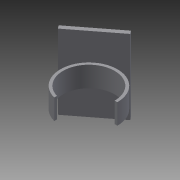
# Autodesk Inventor part: Clip
Saved by Autodesk Inventor 2015 (Build 190159000, 159)
## iProperties
Created: 2018-12-12
Part Number: Clip
Material: Generic
Document SubType Name: Modeling
Designer: 579494
Density: 1 g/cm^3
Appearance: Default
Author: 579494
Autodesk Inventor part; units mm, degrees
ref_plane "YZ Plane" through (0, 0, 0) normal (1, 0, 0) x (0, 1, 0)
ref_plane "XZ Plane" through (0, 0, 0) normal (0, 1, 0) x (-1, 0, 0)
ref_plane "XY Plane" through (0, 0, 0) normal (0, 0, 1) x (1, 0, 0)
sketch "Sketch1" plane through (0, 0, 0) normal (0, 0, 1) x (1, 0, 0)
  arc A0 (19, 0) -> (-5.2482, -18.2608) centre (0, 0) ccw
  line L0 (-5.2482, -18.2608) -> (-5.2482, -20.2608)
  line L1 (19, 0) -> (21, 0)
  arc A1 (21, 0) -> (-5.2482, -20.2608) centre (0.0001, 0.0728) ccw
  line L2 (-12.8316, 16.6965) -> (2.2089, 28.3061)
  line L3 (2.2089, 28.3061) -> (-12.8316, 16.6965)
  line L4 (-12.8316, 16.6965) -> (-27.8721, 5.0869)
  line L5 (-27.8721, 5.0869) -> (-29.7052, 7.4617)
  line L6 (-29.7052, 7.4617) -> (0.3758, 30.681)
  line L7 (0.3758, 30.681) -> (2.2089, 28.3061)
  point P0 (0, 0)
  dimension "d1" = 19
  dimension "d2" = 2
  dimension "d3" = 2
  dimension "d4" = 21
  dimension "d5" = 19
  dimension "d6" = 19
  dimension "d7" = 3
  constraints: 16 end point, 5 point on circle, 2 centre point, 2 perpendicular, 1 collinear, 1 horizontal, 1 point on line, 1 vertical
  measures "d1" radius of A0
  measures "d2" distance of L0.start L0.end
  measures "d3" distance of L1.start L1.end
  measures "d4" radius of A1
  measures "d5" distance of L2.start L2.end
  measures "d6" distance of L2.start L4.end
  measures "d7" distance of L4.end L5.end
extrude "Extrusion1" add sketch "Sketch1" along normal blind 15
sketch "Sketch2" plane through (0, 0, 0) normal (0, 0, -1) x (-1, 0, 0)
  line L0 (29.7052, 7.4617) -> (-0.3758, 30.681)
  line L1 (-0.3758, 30.681) -> (29.7052, 7.4617) projected
  line L2 (-0.3758, 30.681) -> (-2.2089, 28.3061)
  line L3 (-2.2089, 28.3061) -> (27.8721, 5.0869)
  line L4 (27.8721, 5.0869) -> (29.7052, 7.4617)
  point P0 (0, 0)
  constraints: 8 end point, 3 perpendicular, 1 collinear
extrude "Extrusion2" add sketch "Sketch2" along normal blind 20
sketch "Sketch3" plane through (0, 0, 15) normal (0, 0, 1) x (1, 0, 0)
  line L0 (0.3758, 30.681) -> (2.2089, 28.3061)
  line L1 (2.2089, 28.3061) -> (0.3758, 30.681) projected
  line L2 (2.2089, 28.3061) -> (-27.8721, 5.0869)
  line L3 (-27.8721, 5.0869) -> (-12.8316, 16.6965) projected
  line L4 (-27.8721, 5.0869) -> (-29.7052, 7.4617)
  line L5 (-29.7052, 7.4617) -> (0.3758, 30.681)
  point P0 (0, 0)
  constraints: 8 end point, 2 collinear, 2 perpendicular
extrude "Extrusion3" add sketch "Sketch3" along normal blind 20
body "Solid1"
